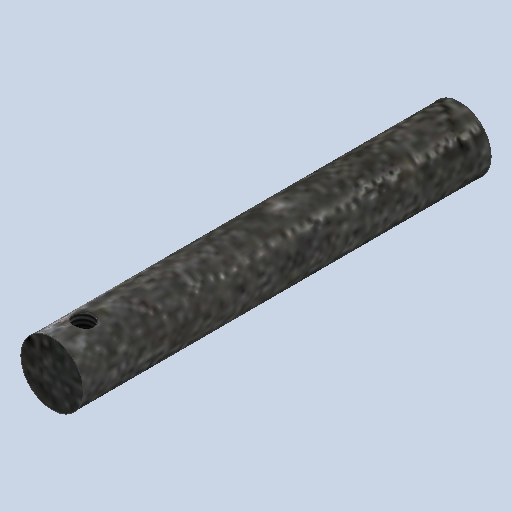
# Autodesk Inventor part: GEARBOX_SHAFT3
Saved by Autodesk Inventor 2023 (Build 270158000, 158)
## iProperties
Created: 2023-05-28
Part Number: GEARBOX_SHAFT3
Material: Steel
Document SubType Name: Modeling
Designer: 310611102
Density: 7.85 g/cm^3
Appearance: Plate
Mass: 39.7336 g
Surface Area: 22.4991 cm^2
Volume: 5.06161 cm^3
Author: 310611102
Autodesk Inventor part; units mm, degrees
ref_plane "YZ Plane" through (0, 0, 0) normal (1, 0, 0) x (0, 1, 0)
ref_plane "XY Plane" through (0, 0, 0) normal (0, 0, 1) x (1, 0, 0)
sketch "Sketch1" plane through (0, 0, 0) normal (0, 0, 1) x (1, 0, 0)
  circle A0 centre (0, 0) radius 5
  dimension "d0" = 10
  constraints: 1 centre point, 1 coincident
  measures "d0" diameter of A0
extrude "Extrusion1" add sketch "Sketch1" along normal blind 65
ref_plane "Work Plane1" through (0, 5, 0) normal (0, 1, 0) x (-1, 0, 0)
sketch "Sketch3" plane through (0, 5, 0) normal (0, 1, 0) x (-1, 0, 0)
  line L0 (5, 65) -> (-5, 65) projected
  point P0 (0, 0)
  point P1 (0, 60)
  point P2 (0, 65)
  dimension "d8" = 5
  constraints: 1 midpoint, 1 vertical alignment
  measures "d8" distance from line of L0 point (0, 60)
hole "Hole1" at (0, 5, 60) direction (0, -1, 0) diameter 3.242 depth 5 tip angle 118 thread size "M4x0.7" class "6H" standard "ISO Metric profile"
sketch "Sketch2" plane through (0, 0, 65) normal (0, 0, 1) x (1, 0, 0)
  line L0 (-2, 12.2946) -> (2, 12.2946)
  line L1 (2, 12.2946) -> (2, 3)
  line L2 (2, 3) -> (-2, 3)
  line L3 (-2, 3) -> (-2, 12.2946)
  line L4 (-2, 12.2946) -> (2, 3) construction
  line L5 (2, 12.2946) -> (-2, 3) construction
  circle A0 centre (0, 0) radius 5 projected
  point P0 (0, 7.6473)
  point P1 (0, 5)
  dimension "d4" = 4
  dimension "d7" = 2
  constraints: 12 end point, 3 vertical alignment, 2 midpoint, 2 parallel, 1 horizontal, 1 perpendicular, 1 other
  measures "d4" distance of L0.start L0.end
  measures "d7" distance from line of L2 point (0, 5)
body "Solid1"
